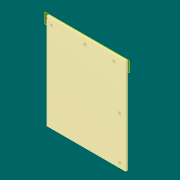
# Autodesk Inventor part: Lado izquierdo
Saved by Autodesk Inventor 2019 (Build 230136000, 136)
## iProperties
Created: 2025-01-01
Part Number: Lado izquierdo
Material: Nylon 6/6
Document SubType Name: Modeling
Designer: Familia CS
Density: 1.13 g/cm^3
Appearance: Nylon 6
Author: Familia CS
Autodesk Inventor part; units mm, degrees
ref_plane "YZ Plane" through (0, 0, 0) normal (1, 0, 0) x (0, 1, 0)
ref_plane "XZ Plane" through (0, 0, 0) normal (0, 1, 0) x (-1, 0, 0)
ref_plane "XY Plane" through (0, 0, 0) normal (0, 0, 1) x (1, 0, 0)
ref_plane "Work Plane1" through (0, 0, 0) normal (0, 0, 1) x (1, 0, 0)
sketch "Sketch1" plane through (0, 0, 0) normal (0, 0, 1) x (1, 0, 0)
  line L0 (0, 2) -> (80.5, 2) projected
  line L1 (0, -8) -> (0, 2) projected
  line L2 (82.5, 2) -> (82.5, -98) projected
  line L3 (82.5, -98) -> (72.5, -98) projected
  circle A0 centre (76.5, -93) radius 0.75 projected
  circle A1 centre (76.5, -48) radius 0.75 projected
  circle A2 centre (70.5, -4) radius 0.75 projected
  circle A3 centre (40.25, -4) radius 0.75 projected
  circle A4 centre (5, -4) radius 0.75 projected
  line L4 (0, 2) -> (82.5, 2)
  line L5 (82.5, 2) -> (82.5, -98)
  line L6 (82.5, -98) -> (0, -98)
  line L7 (0, -98) -> (0, 2)
  point P0 (0, 0)
  constraints: 8 end point, 2 parallel, 1 horizontal, 1 perpendicular
extrude "Extrusion1" add sketch "Sketch1" along normal blind 2
sketch "Sketch2" plane through (0, 0, 2) normal (0, 0, 1) x (1, 0, 0)
  circle A0 centre (76.5, -93) radius 0.75 projected
  circle A1 centre (76.5, -93) radius 1.25
  circle A2 centre (76.5, -48) radius 0.75 projected
  circle A3 centre (76.5, -48) radius 1.25
  circle A4 centre (70.5, -4) radius 0.75 projected
  circle A5 centre (70.5, -4) radius 1.25
  circle A6 centre (40.25, -4) radius 0.75 projected
  circle A7 centre (40.25, -4) radius 1.25
  circle A8 centre (5, -4) radius 0.75 projected
  circle A9 centre (5, -4) radius 1.25
  point P0 (0, 0)
  dimension "d2" = 2.5
  dimension "d3" = 2.5
  dimension "d4" = 2.5
  dimension "d5" = 2.5
  dimension "d6" = 2.5
  constraints: 5 centre point, 5 coincident
  measures "d2" diameter of A1
  measures "d3" diameter of A3
  measures "d4" diameter of A5
  measures "d5" diameter of A7
  measures "d6" diameter of A9
extrude "Extrusion2" cut sketch "Sketch2" against normal blind 2
sketch "Sketch3" plane through (0, -98, 0) normal (-1, 0, 0) x (0, 0, 1)
  line L0 (0, 45) -> (-5, 45) projected
  line L1 (0, 55) -> (-5, 55) projected
  line L2 (0, 45) -> (-8, 45)
  line L3 (-8, 45) -> (-8, 55)
  line L4 (-8, 55) -> (0, 55)
  line L5 (0, 55) -> (0, 45)
  circle A0 centre (-4, 50) radius 0.75
  point P0 (0, 98)
  dimension "d9" = 8
  dimension "d10" = 10
  dimension "d11" = 8
  dimension "d13" = 1.5
  constraints: 8 end point, 1 centre point, 1 horizontal, 1 perpendicular
  measures "d9" distance of L0.start L2.end
  measures "d10" distance of L2.end L3.end
  measures "d11" distance of L3.end L1.start
  measures "d13" diameter of A0
extrude "Extrusion3" add sketch "Sketch3" against normal blind 5
sketch "Sketch4" plane through (0, -98, 2) normal (-1, 0, 0) x (0, 0, 1)
  line L0 (-2, 0) -> (0, 0) projected
  line L1 (-2, 0) -> (-10, 0)
  line L2 (-10, 0) -> (-10, 10)
  line L3 (-10, 10) -> (-2, 10)
  line L4 (-2, 10) -> (-2, 0)
  circle A0 centre (-6, 5) radius 0.75
  point P0 (-2, 98)
  dimension "d16" = 8
  dimension "d17" = 10
  dimension "d19" = 1.5
  constraints: 8 end point, 2 parallel, 1 centre point, 1 horizontal, 1 perpendicular
  measures "d16" distance of L2.end L3.end
  measures "d17" distance of L1.end L2.end
  measures "d19" diameter of A0
extrude "Extrusion4" add sketch "Sketch4" against normal blind 5
sketch "Sketch5" plane through (0, -98, 2) normal (0, -1, 0) x (1, 0, 0)
  line L0 (82.5, -2) -> (5, -2) projected
  line L1 (5, -2) -> (15, -2)
  line L2 (15, -2) -> (15, -10)
  line L3 (15, -10) -> (5, -10)
  line L4 (5, -10) -> (5, -2)
  circle A0 centre (10, -6) radius 0.75
  line L5 (45.25, -2) -> (45.25, -7) projected
  line L6 (35.25, -2) -> (35.25, -7) projected
  line L7 (35.25, -2) -> (45.25, -2)
  line L8 (45.25, -2) -> (45.25, -10)
  line L9 (45.25, -10) -> (35.25, -10)
  line L10 (35.25, -10) -> (35.25, -2)
  circle A1 centre (40.25, -6) radius 0.75
  point P0 (0, -2)
  dimension "d22" = 10
  dimension "d23" = 8
  dimension "d25" = 1.5
  dimension "d27" = 1.5
  constraints: 16 end point, 4 parallel, 2 centre point, 2 horizontal, 2 perpendicular
  measures "d22" distance of L2.end L3.end
  measures "d23" distance of L1.end L2.end
  measures "d25" diameter of A0
  measures "d27" diameter of A1
extrude "Extrusion5" add sketch "Sketch5" against normal blind 5
sketch "Sketch6" plane through (0, 0, 2) normal (0, 0, 1) x (1, 0, 0)
  point P0 (0, 0)
sketch "Sketch7" plane through (0, 0, 2) normal (0, 0, 1) x (1, 0, 0)
  point P0 (0, 0)
sketch "Sketch8" plane through (0, -53, -8) normal (0, 0, -1) x (-1, 0, 0)
  line L0 (-5, 10) -> (0, 10) projected
  line L1 (0, 0) -> (0, 10) projected
  line L2 (-5, 10) -> (0, 10)
  line L3 (0, 10) -> (0, 0)
  line L4 (0, 0) -> (-5, 0)
  line L5 (-5, 0) -> (-5, 10)
  point P0 (0, 53)
  constraints: 8 end point, 2 parallel, 1 horizontal, 1 perpendicular
extrude "Extrusion6" cut sketch "Sketch8" against normal blind 8
sketch "Sketch9" plane through (0, 0, 0) normal (0, 0, -1) x (-1, 0, 0)
  circle A0 centre (-76.5, -48) radius 1.25 projected
  line L0 (0, 2) -> (0, -98) projected
  line L1 (0, -53) -> (0, -63)
  line L2 (0, -63) -> (-8, -63)
  line L3 (-8, -63) -> (-8, -53)
  line L4 (-8, -53) -> (0, -53)
  point P0 (0, 0)
  dimension "d33" = 10
  dimension "d34" = 8
  dimension "d35" = 10
  constraints: 8 end point, 2 perpendicular, 2 point on line
  measures "d33" distance of L1.start L1.end
  measures "d34" distance of L1.end L2.end
  measures "d35" distance of L2.end L3.end
extrude "Extrusion7" add sketch "Sketch9" along normal blind 8 contours L0 L2 L3 L4
sketch "Sketch10" plane through (0, 0, -8) normal (0, 0, -1) x (-1, 0, 0)
  line L0 (0, -88) -> (0, -63) projected
  line L1 (-8, -53) -> (0, -53)
  line L2 (0, -53) -> (0, -63)
  line L3 (0, -63) -> (-8, -63)
  line L4 (-8, -63) -> (-8, -53)
  point P0 (0, 0)
  constraints: 8 end point, 2 parallel, 1 horizontal, 1 perpendicular
extrude "Extrusion8" cut sketch "Sketch10" against normal blind 8
sketch "Sketch11" plane through (0, 0, 0) normal (0, 0, -1) x (-1, 0, 0)
  circle A0 centre (-76.5, -48) radius 1.25 projected
  line L0 (0, -48) -> (0, -33)
  line L1 (0, 2) -> (0, -98) projected
  line L2 (0, -33) -> (-8, -33)
  line L3 (-8, -33) -> (-8, -43)
  line L4 (-8, -43) -> (0, -43)
  point P0 (0, 0)
  dimension "d42" = 15
  dimension "d43" = 8
  dimension "d44" = 10
  constraints: 8 end point, 2 perpendicular, 2 point on line, 1 horizontal
  measures "d42" distance of L0.start L0.end
  measures "d43" distance of L0.end L2.end
  measures "d44" distance of L2.end L3.end
extrude "Extrusion9" add sketch "Sketch11" along normal blind 8 contours L4 L3 L2 L0
sketch "Sketch12" plane through (0, 0, -8) normal (0, 0, -1) x (-1, 0, 0)
  point P0 (0, 0)
sketch "Sketch13" plane through (0, -98, 2) normal (-1, 0, 0) x (0, 0, 1)
  point P0 (-2, 98)
sketch "Sketch14" plane through (0, -98, 2) normal (-1, 0, 0) x (0, 0, 1)
  line L0 (-10, 65) -> (-10, 55) projected
  circle A0 centre (-6, 60) radius 0.75
  point P0 (-2, 98)
  dimension "d50" = 1.5
  constraints: 1 centre point
  measures "d50" diameter of A0
extrude "Extrusion10" cut sketch "Sketch14" against normal blind 8
body "Solid1"
